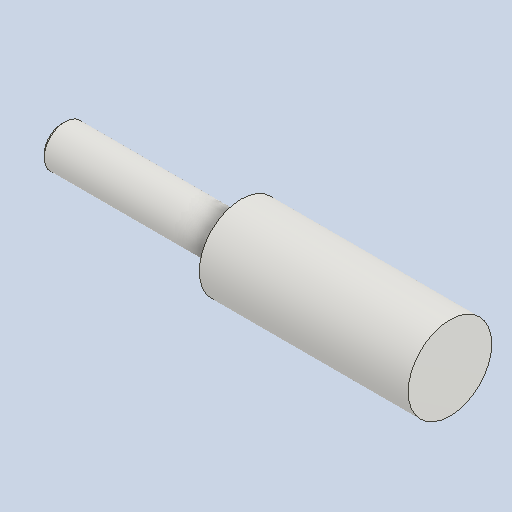
# Autodesk Inventor part: Shaft
Saved by Autodesk Inventor 2024 (Build 280153000, 153)
## iProperties
Created: 2023-09-05
Part Number: Shaft
Material: Steel
Document SubType Name: Modeling
Designer: Pintu
Density: 1 g/cm^3
Appearance: Steel
CustomPartVersion: 1
Author: Pintu
Length: 65.000 mm
Autodesk Inventor part; units mm, degrees
ref_plane "Start Plane" through (0, 0, 0) normal (1, 0, 0) x (0, 1, 0)
ref_plane "XZ Plane" through (0, 0, 0) normal (0, 1, 0) x (-1, 0, 0)
ref_plane "XY Plane" through (0, 0, 0) normal (0, 0, 1) x (1, 0, 0)
sketch "Main Sketch" plane through (0, 0, 0) normal (0, 0, 1) x (1, 0, 0)
  line L0 (0, 0) -> (65, 0)
  line L1 (0, 0) -> (0, 3.5)
  line L2 (0, 3.5) -> (30, 3.5)
  line L3 (30, 3.5) -> (30, 7)
  line L4 (65, 7) -> (65, 0)
  line L5 (30, 7) -> (65, 7)
  dimension "d3" = 7
  dimension "d4" = 14
  constraints: 12 end point, 4 horizontal, 3 vertical
  measures "d3" diameter of L2 L0
  measures "d4" diameter of L5 L0
revolve "Revolution1" add sketch "Main Sketch" angle 360 about axis through (0, 0, 0) along (1, 0, 0)
chamfer "Chamfer1" distance 0.5 angle 45 1 edges at (0, -3.5, 0) measured on face at (0.5, -3.5, 0)
equation "\"Length\" = 65"
body "Solid1"
